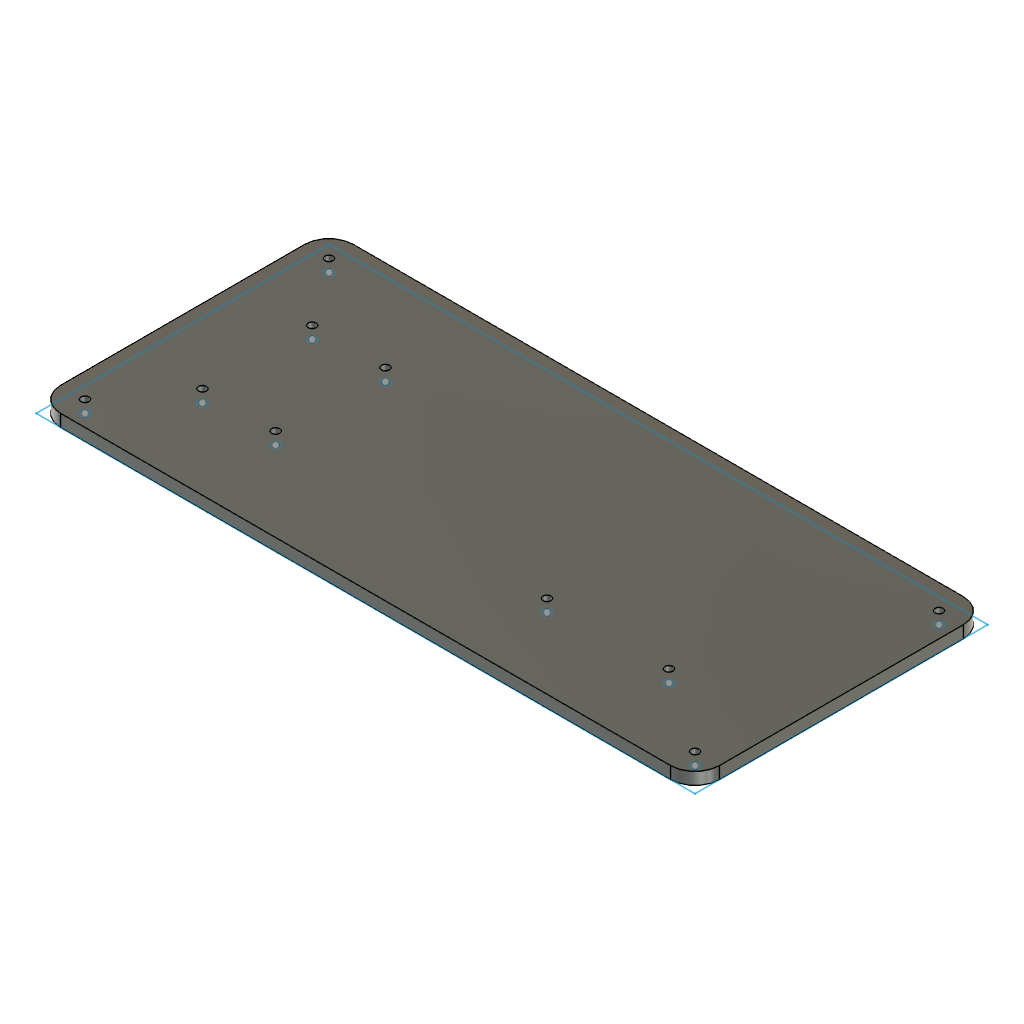
Seminaire_FISA-A3_plaque_20260907 (Autodesk Fusion 360 design; units mm, degrees)
part number: 2026-09-07-10-20-51-535
Autodesk Fusion 360 part; units mm, degrees
sketch "Esquisse2" plane through (0, 0, 0) normal (0, 0, 1) x (1, 0, 0)
  line L0 (-20.3219, 27.194) -> (249.6781, 27.194)
  line L1 (249.6781, 27.194) -> (249.6781, -92.806)
  line L2 (249.6781, -92.806) -> (-20.3219, -92.806)
  line L3 (-20.3219, -92.806) -> (-20.3219, 27.194)
  circle A0 centre (-10.3219, 17.194) radius 1.65
  circle A1 centre (-10.3219, -82.806) radius 1.65
  circle A2 centre (239.6781, 17.194) radius 1.65
  circle A3 centre (239.6781, -82.806) radius 1.65
  circle A4 centre (10, -10) radius 1.65
  circle A5 centre (40, -10) radius 1.65
  circle A6 centre (10, -55) radius 1.65
  circle A7 centre (40, -55) radius 1.65
  circle A8 centre (155, -58.806) radius 1.65
  circle A9 centre (205, -58.806) radius 1.65
  dimension "d1" = 120
  dimension "d2" = 270
  dimension "d20" = 3.3
  dimension "d21" = 10
  dimension "d22" = 10
  dimension "d23" = 3.3
  dimension "d24" = 10
  dimension "d25" = 10
  dimension "d26" = 3.3
  dimension "d27" = 10
  dimension "d28" = 10
  dimension "d29" = 3.3
  dimension "d30" = 10
  dimension "d31" = 10
  dimension "d32" = 3.3
  dimension "d33" = 3.3
  dimension "d34" = 45
  dimension "d35" = 3.3
  dimension "d36" = 30
  dimension "d37" = 3.3
  dimension "d38" = 30
  dimension "d39" = 3.3
  dimension "d40" = 3.3
  dimension "d49" = 34
  dimension "d50" = 115
  dimension "d53" = 34
  dimension "d54" = 50
  constraint horizontal L0
  constraint vertical L1
  constraint horizontal L2
  constraint vertical L3
  measures "d1" distance of L0.start L2.end
  measures "d2" distance of L0.start L0.end
  measures "d20" diameter of A0
  measures "d21" distance of L0 A0.centre
  measures "d22" distance of L3 A0.centre
  measures "d23" diameter of A1
  measures "d24" distance of L2 A1.centre
  measures "d25" distance of L3 A1.centre
  measures "d26" diameter of A2
  measures "d27" distance of L0 A2.centre
  measures "d28" distance of L1 A2.centre
  measures "d29" diameter of A3
  measures "d30" distance of L1 A3.centre
  measures "d31" distance of L2 A3.centre
  measures "d32" diameter of A4
  measures "d33" diameter of A6
  measures "d34" distance of A4.centre A6.centre
  measures "d35" diameter of A5
  measures "d36" distance of A5.centre A4.centre
  measures "d37" diameter of A7
  measures "d38" distance of A7.centre A6.centre
  measures "d39" diameter of A8
  measures "d40" diameter of A9
  measures "d49" distance of L2 A8.centre
  measures "d50" horizontal distance of A7.centre A8.centre
  measures "d53" distance of L2 A9.centre
  measures "d54" distance of A8.centre A9.centre
extrude "Extrusion5" add sketch "Esquisse2" along normal blind 5
fillet "Congé1" radius 10 4 edges at (-20.3219, -92.806, 2.5) (249.6781, -92.806, 2.5) (249.6781, 27.194, 2.5) (-20.3219, 27.194, 2.5)
equation "d3 = 3.30 mm"
equation "d10 = 3.3 mm"
equation "d33 = d3"
equation "d35 = d3"
equation "d37 = d3"
equation "d40 = d10"
